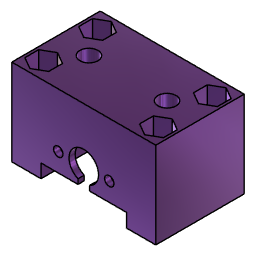
Motor Box 180 v11 (Autodesk Fusion 360 design; units mm, degrees)
Autodesk Fusion 360 part; units mm, degrees
sketch "Main" plane through (0, 0, 0) normal (0, 0, 1) x (1, 0, 0)
  line L0 (0, 0) -> (35, 0)
  line L1 (35, 0) -> (35, 21.5)
  line L2 (35, 21.5) -> (0, 21.5)
  line L3 (0, 21.5) -> (0, 0)
  dimension "d7" = 21.5
  dimension "d8" = 35
  constraint horizontal L0
  constraint vertical L1
  constraint horizontal L2
  constraint vertical L3
  constraint coincident L0.start L3.end
  measures "d7" distance of L0.end L1.end
  measures "d8" distance of L1.end L2.end
extrude "Extrude1" add sketch "Main" along normal blind 21
sketch "Cavidade principal" plane through (0, 0, 0) normal (0, 0, -1) x (1, 0, 0)
  line L0 (0, 0) -> (0, -21.5)
  line L1 (0, -21.5) -> (35, -21.5)
  line L2 (35, -21.5) -> (35, 0)
  line L3 (35, 0) -> (0, 0)
  line L4 (7.1, 0) -> (27.9, 0)
  line L5 (27.9, 0) -> (27.9, -22)
  line L6 (27.9, -22) -> (7.1, -22)
  line L7 (7.1, -22) -> (7.1, 0)
  dimension "d3" = 7.1
  dimension "d4" = 7.1
  dimension "d12" = 22
  constraint horizontal L4
  constraint vertical L5
  constraint horizontal L6
  constraint vertical L7
  constraint coincident L3 L4.start
  measures "d3" distance of L0 L7
  measures "d4" distance of L2 L5
  measures "d12" distance of L4 L6
extrude "Extrude2" cut sketch "Cavidade principal" against normal blind 15.3 contours L1 L3 L4 L5 L7 | L1 L5 L6 L7
sketch "Batente" plane through (0, 0, 15.3) normal (0, 0, -1) x (1, 0, 0)
  line L0 (27.9, -21.5) -> (27.9, 0)
  line L1 (27.9, 0) -> (7.1, 0)
  line L2 (7.1, 0) -> (7.1, -21.5)
  line L3 (7.1, 0) -> (27.9, 0)
  line L4 (27.9, 0) -> (27.9, -1.5)
  line L5 (27.9, -1.5) -> (7.1, -1.5)
  line L6 (7.1, -1.5) -> (7.1, 0)
  line L7 (7.1, -21.5) -> (27.9, -21.5)
  dimension "d9" = 1.5
  constraint horizontal L3
  constraint vertical L4
  constraint horizontal L5
  constraint vertical L6
  constraint coincident L0 L4.end
  constraint coincident L1.end L2.start
  measures "d9" distance of L0.end L4.end
extrude "Extrude3" add sketch "Batente" along normal blind 12 contours L0 L1 L2 L3 L4 L5 L6
sketch "Curvatura" plane through (0, 21.5, 0) normal (0, 1, 0) x (-1, 0, 0)
  line L0 (-27.9, 0) -> (-27.9, 15.3)
  line L1 (-27.9, 15.3) -> (-7.1, 15.3)
  line L2 (-7.1, 15.3) -> (-7.1, 0)
  line L3 (-7.1, 0) -> (0, 0)
  line L4 (0, 0) -> (0, 21)
  line L5 (0, 21) -> (-35, 21)
  line L6 (-35, 21) -> (-35, 0)
  line L7 (-35, 0) -> (-27.9, 0)
  line L8 (-7.1, 15.3) -> (-7.1, 8.3)
  line L9 (-7.1, 15.3) -> (-10.2, 15.3)
  line L10 (-27.9, 15.3) -> (-27.9, 8.3)
  line L11 (-27.9, 15.3) -> (-24.8, 15.3)
  arc A0 (-24.8, 15.3) -> (-27.9, 8.3) centre (-16.2213, 7.3144) ccw
  arc A1 (-10.2, 15.3) -> (-7.1, 8.3) centre (-18.7405, 7.3313) cw
  dimension "d13" = 7
  dimension "d14" = 3.1
  dimension "d15" = 7
  dimension "d16" = 3.1
  constraint coincident L1.end L2.start
  constraint parallel L1 L9
  constraint coincident L0.end L1.start
  constraint coincident L0 L10.end
  constraint perpendicular L1 L10
  constraint coincident L1 L11.end
  constraint perpendicular L10 L11
  constraint coincident L2 L8.end
  constraint coincident L9.end A1.start
  constraint coincident L8.end A1.end
  measures "d13" vertical distance of L1.end L8.end
  measures "d14" distance of L1.end L9.end
  measures "d15" distance of L0.end L10.end
  measures "d16" distance of L0.end L11.end
extrude "Extrude4" add sketch "Curvatura" against normal up to surface (20 mm away) contours L0 L1 L2 L3 L4 L5 L6 L7 L8 L9 L10 L11 | L0 L1 L10 L11 A0
sketch "Furos" plane through (0, 0, 21) normal (0, 0, 1) x (-1, 0, 0)
  line L0 (0, -21.5) -> (0, 0)
  line L1 (0, 0) -> (-35, 0)
  line L2 (-35, 0) -> (-35, -21.5)
  line L3 (-35, -21.5) -> (0, -21.5)
  line L4 (-7.1, -21.5) -> (0, -21.5) construction
  line L5 (0, 0) -> (-7.1, 0) construction
  line L6 (-3.55, -21.5) -> (-3.55, 0) construction
  line L7 (-35, -21.5) -> (-27.9, -21.5) construction
  line L8 (-27.9, 0) -> (-35, 0) construction
  line L9 (-31.45, -21.5) -> (-31.45, 0) construction
  line L10 (0, -17.3) -> (-35, -17.3) construction
  line L11 (0, -4.2) -> (-35, -4.2) construction
  circle A0 centre (-3.55, -17.3) radius 1.6
  circle A1 centre (-3.55, -4.2) radius 1.6
  circle A2 centre (-31.45, -17.3) radius 1.6
  circle A3 centre (-31.45, -4.2) radius 1.6
  dimension "d19" = 4.2
  dimension "d20" = 4.2
  dimension "d21" = 3.2
  dimension "d22" = 3.2
  dimension "d23" = 3.2
  dimension "d24" = 3.2
  constraint midpoint L4 L6.start
  constraint midpoint L5 L6.end
  constraint midpoint L7 L9.start
  constraint midpoint L8 L9.end
  constraint coincident L0 L10.start
  constraint coincident L2 L10.end
  constraint perpendicular L2 L10
  constraint coincident L0 L11.start
  constraint coincident L2 L11.end
  constraint perpendicular L2 L11
  constraint coincident L6 A0.centre
  constraint coincident L10 A0.centre
  constraint coincident L11 A1.centre
  constraint coincident L6 A1.centre
  constraint coincident L10 A2.centre
  constraint coincident L9 A2.centre
  constraint coincident L11 A3.centre
  constraint coincident L9 A3.centre
  measures "d19" distance of L3 L10
  measures "d20" distance of L1 L11
  measures "d21" diameter of A0
  measures "d22" diameter of A1
  measures "d23" diameter of A2
  measures "d24" diameter of A3
extrude "Extrude5" cut sketch "Furos" against normal blind 21 contours A0 | A1 | A2 | A3
sketch "Rebaixo hexagonal furos" plane through (0, 0, 21) normal (0, 0, 1) x (-1, 0, 0)
  circle A0 centre (-3.55, -17.3) radius 1.6
  circle A1 centre (-31.45, -4.2) radius 1.6
  circle A2 centre (-3.55, -4.2) radius 1.6
  circle A3 centre (-31.45, -17.3) radius 1.6
  line L0 (0, -21.5) -> (0, 0)
  line L1 (0, 0) -> (-35, 0)
  line L2 (-35, 0) -> (-35, -21.5)
  line L3 (-35, -21.5) -> (0, -21.5)
  line L4 (-6.45, -18.9743) -> (-3.55, -20.6486)
  line L5 (-3.55, -20.6486) -> (-0.65, -18.9743)
  line L6 (-0.65, -18.9743) -> (-0.65, -15.6257)
  line L7 (-0.65, -15.6257) -> (-3.55, -13.9514)
  line L8 (-3.55, -13.9514) -> (-6.45, -15.6257)
  line L9 (-6.45, -15.6257) -> (-6.45, -18.9743)
  line L10 (-6.45, -5.8743) -> (-3.55, -7.5486)
  line L11 (-3.55, -7.5486) -> (-0.65, -5.8743)
  line L12 (-0.65, -5.8743) -> (-0.65, -2.5257)
  line L13 (-0.65, -2.5257) -> (-3.55, -0.8514)
  line L14 (-3.55, -0.8514) -> (-6.45, -2.5257)
  line L15 (-6.45, -2.5257) -> (-6.45, -5.8743)
  line L16 (-34.35, -18.9743) -> (-31.45, -20.6486)
  line L17 (-31.45, -20.6486) -> (-28.55, -18.9743)
  line L18 (-28.55, -18.9743) -> (-28.55, -15.6257)
  line L19 (-28.55, -15.6257) -> (-31.45, -13.9514)
  line L20 (-31.45, -13.9514) -> (-34.35, -15.6257)
  line L21 (-34.35, -15.6257) -> (-34.35, -18.9743)
  line L22 (-34.35, -5.8743) -> (-31.45, -7.5486)
  line L23 (-31.45, -7.5486) -> (-28.55, -5.8743)
  line L24 (-28.55, -5.8743) -> (-28.55, -2.5257)
  line L25 (-28.55, -2.5257) -> (-31.45, -0.8514)
  line L26 (-31.45, -0.8514) -> (-34.35, -2.5257)
  line L27 (-34.35, -2.5257) -> (-34.35, -5.8743)
  point P0 (-3.55, -17.3)
  point P1 (-3.55, -4.2)
  point P2 (-31.45, -17.3)
  point P3 (-31.45, -4.2)
  dimension "d27" = 2.9
  dimension "d30" = 2.9
  dimension "d31" = 2.9
  dimension "d32" = 2.9
  constraint coincident P0 A0.centre
  constraint coincident P1 A2.centre
  constraint coincident P2 A3.centre
  constraint coincident P3 A1.centre
  constraint vertical L12
  constraint vertical L18
  constraint vertical L24
  constraint vertical L6
  measures "d27" distance of P0 L9
  measures "d30" distance of P1 L15
  measures "d31" distance of P2 L21
  measures "d32" distance of P3 L27
extrude "Extrude6" cut sketch "Rebaixo hexagonal furos" against normal blind 14.5 contours L4 L5 L6 L7 L8 L9 | L10 L11 L12 L13 L14 L15 | L16 L17 L18 L19 L20 L21 | L22 L23 L24 L25 L26 L27
extrude "Extrude14" add sketch "Curvatura" against normal up to surface (21.5 mm away) contours L1 L2 L8 L9 A1
sketch "Sketch8" plane through (0, 0, 21) normal (0, 0, 1) x (-1, 0, 0)
  line L0 (-3.55, -7.5486) -> (-6.45, -5.8743)
  line L1 (-6.45, -5.8743) -> (-6.45, -2.5257)
  line L2 (-6.45, -2.5257) -> (-3.55, -0.8514)
  line L3 (-3.55, -0.8514) -> (-0.65, -2.5257)
  line L4 (-0.65, -2.5257) -> (-0.65, -5.8743)
  line L5 (-0.65, -5.8743) -> (-3.55, -7.5486)
  line L6 (-31.45, -20.6486) -> (-34.35, -18.9743)
  line L7 (-34.35, -18.9743) -> (-34.35, -15.6257)
  line L8 (-34.35, -15.6257) -> (-31.45, -13.9514)
  line L9 (-31.45, -13.9514) -> (-28.55, -15.6257)
  line L10 (-28.55, -15.6257) -> (-28.55, -18.9743)
  line L11 (-28.55, -18.9743) -> (-31.45, -20.6486)
  line L12 (-3.55, -20.6486) -> (-6.45, -18.9743)
  line L13 (-6.45, -18.9743) -> (-6.45, -15.6257)
  line L14 (-6.45, -15.6257) -> (-3.55, -13.9514)
  line L15 (-3.55, -13.9514) -> (-0.65, -15.6257)
  line L16 (-0.65, -15.6257) -> (-0.65, -18.9743)
  line L17 (-0.65, -18.9743) -> (-3.55, -20.6486)
  line L18 (-31.45, -7.5486) -> (-34.35, -5.8743)
  line L19 (-34.35, -5.8743) -> (-34.35, -2.5257)
  line L20 (-34.35, -2.5257) -> (-31.45, -0.8514)
  line L21 (-31.45, -0.8514) -> (-28.55, -2.5257)
  line L22 (-28.55, -2.5257) -> (-28.55, -5.8743)
  line L23 (-28.55, -5.8743) -> (-31.45, -7.5486)
  line L24 (0, -21.5) -> (0, 0)
  line L25 (0, 0) -> (-35, 0)
  line L26 (-35, 0) -> (-35, -21.5)
  line L27 (-35, -21.5) -> (0, -21.5)
  line L28 (0, -10.75) -> (-35, -10.75) construction
  circle A0 centre (-8, -10.75) radius 2.2
  circle A1 centre (-27, -10.75) radius 2.2
  dimension "d68" = 4.4
  dimension "d69" = 4.4
  dimension "d70" = 8
  dimension "d71" = 8
  constraint midpoint L24 L28.start
  constraint midpoint L26 L28.end
  constraint coincident L28 A0.centre
  constraint coincident L28 A1.centre
  measures "d68" diameter of A0
  measures "d69" diameter of A1
  measures "d70" distance of L24 A0.centre
  measures "d71" distance of L26 A1.centre
extrude "Extrude15" cut sketch "Sketch8" against normal blind 5 contours A0 | A1
sketch "Furos Motor" plane through (0, 0, 0) normal (0, -1, 0) x (1, 0, 0)
  line L0 (27.9, 3.3) -> (27.9, 0)
  line L1 (27.9, 0) -> (35, 0)
  line L2 (35, 0) -> (35, 21)
  line L3 (35, 21) -> (0, 21)
  line L4 (0, 21) -> (0, 0)
  line L5 (0, 0) -> (7.1, 0)
  line L6 (7.1, 0) -> (7.1, 3.3)
  line L7 (7.1, 3.3) -> (27.9, 3.3)
  circle A0 centre (17.5, 7.8) radius 3.6
  line L8 (0, 7.8) -> (35, 7.8) construction
  circle A1 centre (23.7, 7.8) radius 1.15
  circle A2 centre (11.3, 7.8) radius 1.15
  dimension "d74" = 7.2
  dimension "d75" = 17.5
  dimension "d76" = 7.8
  dimension "d79" = 2.3
  dimension "d80" = 6.2
  dimension "d81" = 2.3
  dimension "d82" = 6.2
  constraint coincident L4 L8.start
  constraint coincident L2 L8.end
  constraint perpendicular L2 L8
  constraint coincident A0.centre L8
  constraint coincident L8 A1.centre
  constraint coincident L8 A2.centre
  measures "d74" diameter of A0
  measures "d75" distance of L2 A0.centre
  measures "d76" distance of L1 L8
  measures "d79" diameter of A1
  measures "d80" distance of A0.centre A1.centre
  measures "d81" diameter of A2
  measures "d82" distance of A0.centre A2.centre
extrude "Extrude16" cut sketch "Furos Motor" against normal blind 3 contours A0 | A1 | A2
sketch "Sketch10" plane through (0, 0, 3.3) normal (0, 0, -1) x (1, 0, 0)
  line L0 (7.1, -1.5) -> (27.9, -1.5)
  line L1 (27.9, -1.5) -> (27.9, 0)
  line L2 (27.9, 0) -> (7.1, 0)
  line L3 (7.1, 0) -> (7.1, -1.5)
  line L4 (16.1, 0) -> (18.9, 0)
  line L5 (18.9, 0) -> (18.9, -1.5)
  line L6 (18.9, -1.5) -> (16.1, -1.5)
  line L7 (16.1, -1.5) -> (16.1, 0)
  dimension "d83" = 9
  dimension "d84" = 9
  constraint horizontal L4
  constraint vertical L5
  constraint horizontal L6
  constraint vertical L7
  constraint coincident L0 L5.end
  constraint coincident L2 L4.start
  measures "d83" distance of L3 L7
  measures "d84" distance of L1 L5
extrude "Extrude17" cut sketch "Sketch10" against normal blind 3.5 contours L0 L2 L4 L5 L6 L7
